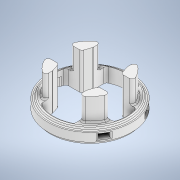
# Autodesk Inventor part: PlanetCarriage
Saved by Autodesk Inventor 2020 (Build 240168000, 168)
## iProperties
Created: 2019-07-19
Part Number: PlanetCarriage
Material: ABS Plastic
Document SubType Name: Modeling
Designer: Connor
Density: 1.06 g/cm^3
Appearance: White
Author: Connor
Autodesk Inventor part; units mm, degrees
ref_plane "YZ Plane" through (0, 0, 0) normal (1, 0, 0) x (0, 1, 0)
ref_plane "XZ Plane" through (0, 0, 0) normal (0, 1, 0) x (-1, 0, 0)
ref_plane "XY Plane" through (0, 0, 0) normal (0, 0, 1) x (1, 0, 0)
sketch "Sketch1" plane through (0, 0, 0) normal (0, 0, 1) x (1, 0, 0)
  line L0 (0, 0) -> (44.323, 0)
  line L1 (44.323, 0) -> (44.323, 3.175)
  line L2 (44.323, 3.175) -> (46.99, 3.175)
  line L3 (46.99, 3.175) -> (46.99, 12.7)
  line L4 (38.1, 15.875) -> (38.1, 41.275)
  line L5 (38.1, 41.275) -> (0, 41.275)
  line L6 (0, 41.275) -> (0, 0)
  line L7 (44.6024, 12.7) -> (42.7693, 15.875)
  line L8 (42.7693, 15.875) -> (38.1, 15.875)
  line L9 (46.99, 12.7) -> (44.6024, 12.7)
  dimension "d0" = 44.323
  dimension "d1" = 3.175
  dimension "d2" = 46.99
  dimension "d3" = 38.1
  dimension "d7" = 12.7
  dimension "d10" = 44.6024
  dimension "d33" = 120
  dimension "d35" = 3.175
  dimension "d46" = 38.1
  constraints: 20 end point, 7 perpendicular, 2 horizontal
  measures "d0" distance between parallel lines of L1 L6
  measures "d1" distance of L0.end L1.end
  measures "d2" distance between parallel lines of L6 L3
  measures "d3" distance between parallel lines of L4 L6
  measures "d7" distance between parallel lines of L0 L9
  measures "d10" distance from line of L6 L7.start
  measures "d33" angle of L9 L7
  measures "d35" distance between parallel lines of L9 L8
  measures "d46" distance between parallel lines of L2 L5
revolve "Revolution1" add sketch "Sketch1" angle 360 about axis through (0, 41.275, 0) along (0, -1, 0)
sketch "Sketch2" plane through (0, 0, 0) normal (0, -1, 0) x (1, 0, 0)
  circle A0 centre (0, 0) radius 41.275
  line L0 (19.05, -36.6159) -> (19.05, 36.6159)
  line L1 (-19.05, -36.6159) -> (-19.05, 36.6159)
  line L2 (39.2726, -12.7) -> (19.05, -12.7)
  line L3 (39.2726, 12.7) -> (19.05, 12.7)
  line L4 (-39.2726, -12.7) -> (-19.05, -12.7)
  line L5 (-39.2726, 12.7) -> (-19.05, 12.7)
  circle A1 centre (30.48, 0) radius 12.7
  circle A2 centre (-30.48, 0) radius 12.7
  line L6 (30.48, 0) -> (0, 0) construction
  line L7 (0, 0) -> (-30.48, 0) construction
  line L8 (-22.352, 12.7) -> (-19.05, 22.8625)
  line L9 (19.05, 22.8625) -> (22.352, 12.7)
  line L10 (19.05, -22.8625) -> (22.352, -12.7)
  line L11 (-22.352, -12.7) -> (-19.05, -22.8625)
  point P0 (-40.5408, -7.7505)
  point P1 (-40.5408, 7.7505)
  point P2 (40.5408, 7.7505)
  point P3 (40.5408, -7.7505)
  dimension "d19" = 82.55
  dimension "d15" = 38.1
  dimension "d36" = 25.4
  dimension "d37" = 60.96
  dimension "d43" = 72
  dimension "d44" = 72
  dimension "d45" = 3.302
  constraints: 24 end point, 12 point on line, 11 equal length, 4 perpendicular, 2 centre point, 2 vertical, 1 coincident, 1 equal radius, 1 horizontal, 1 tangent, 10 other
  measures "d15" distance between parallel lines of L1 L0
  measures "d36" diameter of A1
  measures "d37" distance of L7.end L6.start
  measures "d43" angle of L5 L8
  measures "d44" angle of L3 L9
  measures "d45" distance of L5.end L8.start
extrude "Extrusion1" cut sketch "Sketch2" against normal through all contours A0 A1 L3 | L0 A1 A0 L1 A2 | A0 A1 L0 | A1 L0 L3 | L9 L3 L0 | L0 A1 | L5 A2 A0 | L1 L5 L8 | A0 L2 A1 | A1 L2 L0 | A2 L1 A0 | L5 L1 A2 | L2 L10 L0 | A2 L4 A0 | A2 L1 | A2 L1 L4 | L4 L1 L11
extrude "Extrusion3" cut sketch "Sketch2" against normal blind 9.525 contours A1 A0 | L9 L3 L0 | L1 L5 L8 | A0 A2 | L2 L10 L0 | L4 L1 L11
fillet "Fillet2" radius 3.175 28 edges at (-19.05, 7.9375, 36.6159) (19.05, 7.9375, 36.6159) (-19.05, 7.9375, -36.6159) (19.05, 7.9375, -36.6159) (39.2726, 7.9375, 12.7) (39.2726, 7.9375, -12.7) (-39.2726, 7.9375, -12.7) (-39.2726, 7.9375, 12.7) (19.05, 28.575, -32.9956) (35.921, 28.575, -12.7) (35.921, 28.575, 12.7) (19.05, 28.575, 32.9956) (-35.921, 28.575, 12.7) (-19.05, 28.575, 32.9956) (-35.921, 28.575, -12.7) (-19.05, 28.575, -32.9956) (-22.352, 20.6375, 12.7) (-19.05, 20.6375, 22.8625) (22.352, 20.6375, 12.7) (19.05, 20.6375, 22.8625) (40.5408, 4.7625, 7.7505) (40.5408, 4.7625, -7.7505) (22.352, 20.6375, -12.7) (19.05, 20.6375, -22.8625) (-19.05, 20.6375, -22.8625) (-22.352, 20.6375, -12.7) (-40.5408, 4.7625, 7.7505) (-40.5408, 4.7625, -7.7505)
sketch "Sketch3" plane through (0, 0, 0) normal (0, -1, 0) x (1, 0, 0)
  line L0 (31.75, -19.05) -> (-31.75, -19.05) construction
  line L1 (-31.75, -19.05) -> (-31.75, 19.05) construction
  line L2 (-31.75, 19.05) -> (31.75, 19.05) construction
  line L3 (31.75, 19.05) -> (31.75, -19.05) construction
  line L4 (31.75, -19.05) -> (-31.75, 19.05) construction
  line L5 (31.75, 19.05) -> (-31.75, -19.05) construction
  point P0 (0, 0)
  point P1 (0, 0)
  dimension "d21" = 63.5
  dimension "d22" = 38.1
  constraints: 12 end point, 2 parallel, 1 coincident, 1 horizontal, 1 midpoint, 1 perpendicular
  measures "d21" distance of L0.start L0.end
  measures "d22" distance of L0.end L1.end
hole "Hole1" at (31.75, 0, -19.05) at (-31.75, 0, -19.05) at (-31.75, 0, 19.05) at (31.75, 0, 19.05) direction (0, 1, 0) diameter 5.207 depth 11.1125
sketch "Sketch4" plane through (31.75, 11.1125, -19.05) normal (0, -1, 0) x (1, 0, 0)
  circle A0 centre (0, 0) radius 2.6035 projected
  circle A1 centre (-31.75, 19.05) radius 46.99 projected
  circle A2 centre (-63.5, 38.1) radius 2.6035 construction
  line L0 (0, 0) -> (-63.5, 38.1) construction
  line L1 (-4.8413, 2.9048) -> (0.095, 5.6451)
  line L2 (0.095, 5.6451) -> (4.9363, 2.7403)
  line L3 (4.9363, 2.7403) -> (4.8413, -2.9048)
  line L4 (4.8413, -2.9048) -> (-0.095, -5.6451)
  line L5 (-0.095, -5.6451) -> (-4.9363, -2.7403)
  line L6 (-4.9363, -2.7403) -> (-4.8413, 2.9048)
  line L7 (4.9363, 2.7403) -> (10.8405, -0.8022)
  line L8 (-0.095, -5.6451) -> (5.8092, -9.1876)
  dimension "d30" = 9.779
  constraints: 18 end point, 2 collinear, 2 point on circle, 1 coincident, 1 point on line, 13 other
  measures "d30" distance between parallel lines of L3 L6
extrude "Extrusion2" cut sketch "Sketch4" along normal blind 6.35 contours L8 L4 L3 L7 A1 | L5 L6 L1 L2 L3 L4
mirror "Mirror1" about plane through (0, 0, 0) normal (0, 0, 1) of "Extrusion2"
mirror "Mirror2" about plane through (0, 0, 0) normal (1, 0, 0) of "Extrusion2", "Mirror1"
fillet "Fillet1" radius 1.5875 14 edges at (-42.7693, 15.875, 0) (-44.6024, 12.7, 0) (37.5592, 7.9375, -28.2376) (42.5905, 7.9375, -19.8522) (42.5905, 7.9375, 19.8522) (37.5592, 7.9375, 28.2376) (-37.5592, 7.9375, 28.2376) (-42.5905, 7.9375, 19.8522) (-42.5905, 7.9375, -19.8522) (-37.5592, 7.9375, -28.2376) (-29.7106, 15.875, 23.8514) (29.7106, 15.875, 23.8514) (-29.7106, 15.875, -23.8514) (29.7106, 15.875, -23.8514)
body "Solid1"
